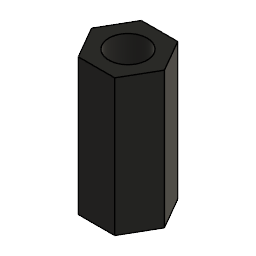
Standoff 15mm_v6 (Autodesk Fusion 360 design; units mm, degrees)
Autodesk Fusion 360 part; units mm, degrees
sketch "Sketch1" plane through (0, 0, 0) normal (0, 0, 1) x (1, 0, 0)
  circle A0 centre (0, 0) radius 2.1
  circle A1 centre (0, 0) radius 3.6
  line L0 (4, 0) -> (2, 3.4641)
  line L1 (2, 3.4641) -> (-2, 3.4641)
  line L2 (-2, 3.4641) -> (-4, 0)
  line L3 (-4, 0) -> (-2, -3.4641)
  line L4 (-2, -3.4641) -> (2, -3.4641)
  line L5 (2, -3.4641) -> (4, 0)
  dimension "d1" = 4.2
  dimension "d2" = 1.5
  constraint coincident A0.centre A1.centre
  constraint concentric A0 A1
  measures "d1" diameter of A0
  measures "d2" distance of A0 A1
extrude "Extrude3" add sketch "Sketch1" against normal blind 12 contours A0 | A1 L0 L1 L2 L3 L4 L5 | A1 L0 L5 | A1 L0 L1 | A1 L4 L5 | A1 L1 L2 | A1 L3 L4 | A1 L2 L3
extrude "Extrude4" cut sketch "Sketch1" along normal blind 3 and the other way blind 3 contours A0
extrude "Extrude5" cut sketch "Sketch1" along normal blind 9 from surface at -17 contours A0
move_face "OffsetFaces1" offset 3 1 faces at (-2.6307, -1.4584, 0)
equation "d9 = -17.00 mm + 5 mm"
